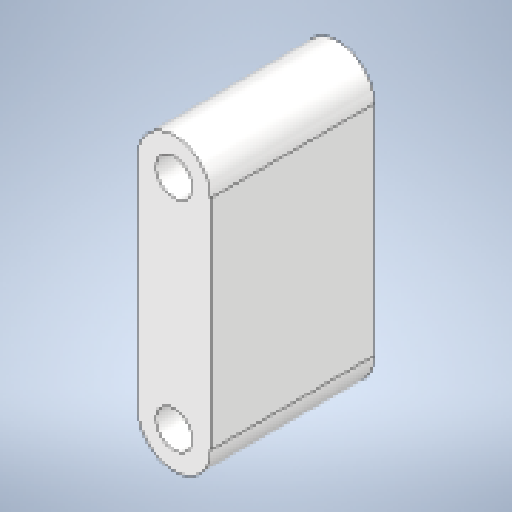
# Autodesk Inventor part: Bracket - 1
Saved by Autodesk Inventor 2023.2 (Build 272271000, 271)
## iProperties
Created: 2024-01-24
Part Number: Bracket - 1
Material: UHMW, White
Document SubType Name: Modeling
Designer: Nathan Cai
Density: 0.94 g/cm^3
Appearance: Smooth - White
Author: Nathan Cai
Autodesk Inventor part; units mm, degrees
ref_plane "YZ Plane" through (0, 0, 0) normal (1, 0, 0) x (0, 1, 0)
ref_plane "XZ Plane" through (0, 0, 0) normal (0, 1, 0) x (-1, 0, 0)
ref_plane "XY Plane" through (0, 0, 0) normal (0, 0, 1) x (1, 0, 0)
sketch "Sketch1" plane through (0, 0, 0) normal (0, 0, 1) x (1, 0, 0)
  line L0 (0, 0) -> (0, -19.05) construction
  line L1 (-3.175, 0) -> (-3.175, -19.05)
  line L2 (3.175, -19.05) -> (3.175, 0)
  arc A0 (3.175, 0) -> (-3.175, 0) centre (0, 0) ccw
  arc A1 (-3.175, -19.05) -> (3.175, -19.05) centre (0, -19.05) ccw
  circle A2 centre (0, 0) radius 1.5875
  circle A3 centre (0, -19.05) radius 1.5875
  point P0 (0, -9.525)
  dimension "d0" = 19.05
  dimension "d1" = 6.35
  dimension "d2" = 3.175
  dimension "d3" = 3.175
  constraints: 8 end point, 4 centre point, 4 point on circle, 4 tangent, 2 coincident, 1 midpoint, 1 parallel, 1 vertical
  measures "d0" distance of L0.start L0.end
  measures "d1" diameter of A1
  measures "d2" diameter of A2
  measures "d3" diameter of A3
extrude "Extrusion1" add sketch "Sketch1" along normal blind 14.2875
body "Solid1"
